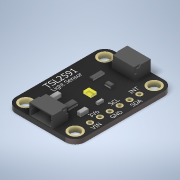
# Autodesk Inventor part: TSL2591
Saved by Autodesk Inventor 2020 (Build 240168000, 168)
## iProperties
Created: 2021-03-24
Part Number: TSL2591
Material: Polyéthylène, densité élevée
Document SubType Name: Modeling
Designer: Charles
Density: 0.952 g/cm^3
Appearance: Lustré - Noir
Author: Charles
Autodesk Inventor part; units mm, degrees
(part 1 of 2)
ref_plane "YZ Plane" through (0, 0, 0) normal (1, 0, 0) x (0, 1, 0)
ref_plane "XZ Plane" through (0, 0, 0) normal (0, 1, 0) x (-1, 0, 0)
ref_plane "XY Plane" through (0, 0, 0) normal (0, 0, 1) x (1, 0, 0)
sketch "Esquisse1" plane through (0, 0, 0) normal (0, 1, 0) x (-1, 0, 0)
  line L0 (0, 0) -> (17.78, 0)
  line L1 (17.78, 0) -> (17.78, -25.4)
  line L2 (17.78, -25.4) -> (0, -25.4)
  line L3 (0, -25.4) -> (0, 0)
  dimension "d0" = 25.4
  dimension "d1" = 17.78
  constraints: 8 end point, 2 parallel, 1 horizontal, 1 perpendicular
  measures "d0" distance of L2.end L0.start
  measures "d1" distance of L1.end L2.end
extrude "Extrusion1" add sketch "Esquisse1" along normal blind 1.2
sketch "Esquisse2" plane through (0, 1.2, 0) normal (0, 1, 0) x (1, 0, 0)
  line L0 (0, 0) -> (0, 25.4) projected
  line L1 (0, 25.4) -> (-17.78, 25.4) projected
  line L2 (0, 0) -> (-17.78, 0)
  line L3 (-17.78, 0) -> (-17.78, 25.4)
  line L4 (-17.78, 25.4) -> (0, 25.4)
  line L5 (0, 25.4) -> (0, 0)
  line L6 (-15.24, 22.86) -> (-15.24, 2.54)
  line L7 (-15.24, 2.54) -> (-2.54, 2.54)
  line L8 (-2.54, 2.54) -> (-2.54, 22.86)
  line L9 (-2.54, 22.86) -> (-15.24, 22.86)
  dimension "d4" = 2.54
  constraints: 16 end point, 4 coincident, 4 parallel, 2 perpendicular, 1 horizontal, 3 other
  measures "d4" distance between parallel lines of L3 L6
hole "Perçage1" at (-15.24, 1.2, -2.54) at (-2.54, 1.2, -2.54) at (-15.24, 1.2, -22.86) at (-2.54, 1.2, -22.86) direction (0, -1, 0) diameter 2.54 end through all
fillet "Congé1" radius 2.54 4 edges at (-17.78, 0.6, 0) (0, 0.6, 0) (0, 0.6, -25.4) (-17.78, 0.6, -25.4)
sketch "Esquisse3" plane through (0, 1.2, 0) normal (0, 1, 0) x (1, 0, 0)
  circle A0 centre (-2.54, 2.54) radius 1.27 projected
  circle A1 centre (-2.54, 22.86) radius 1.27 projected
  line L0 (-2.54, 2.54) -> (-2.54, 22.86)
  circle A2 centre (-2.54, 6.35) radius 0.4
  line L1 (-2.54, 3.81) -> (-4.1087, 3.81)
  circle A3 centre (-2.54, 8.89) radius 0.4
  circle A4 centre (-2.54, 11.43) radius 0.4
  circle A5 centre (-2.54, 13.97) radius 0.4
  circle A6 centre (-2.54, 16.51) radius 0.4
  circle A7 centre (-2.54, 19.05) radius 0.4
  line L2 (-2.54, 21.59) -> (-3.81, 21.59)
  circle A8 centre (-2.54, 6.35) radius 0.75
  circle A9 centre (-2.54, 2.54) radius 1.77
  circle A10 centre (-2.54, 22.86) radius 1.77
  circle A11 centre (-15.24, 22.86) radius 1.27 projected
  circle A12 centre (-15.24, 22.86) radius 1.77
  circle A13 centre (-15.24, 2.54) radius 1.27 projected
  circle A14 centre (-15.24, 2.54) radius 1.77
  circle A15 centre (-2.54, 8.89) radius 0.75
  circle A16 centre (-2.54, 11.43) radius 0.75
  circle A17 centre (-2.54, 13.97) radius 0.75
  circle A18 centre (-2.54, 16.51) radius 0.75
  circle A19 centre (-2.54, 19.05) radius 0.75
  point P0 (0, 0)
  dimension "d13" = 0.8
  dimension "d14" = 2.54
  dimension "d17" = 2.54
  dimension "d23" = 1.5
  dimension "d24" = 3.54
  dimension "d27" = 2.54
  constraints: 16 centre point, 6 end point, 5 coincident, 4 horizontal, 3 point on line, 3 vertical, 2 vertical alignment, 22 other
  measures "d13" diameter of A2
  measures "d14" distance of L1.start A2.centre
  measures "d17" distance of A2.centre A3.centre
  measures "d23" diameter of A8
  measures "d24" diameter of A9
  measures "d27" distance of A8.centre A15.centre
extrude "Extrusion2" cut sketch "Esquisse3" against normal blind 1.2 contours A2 L0 | L0 A2 | A3 L0 | L0 A3 | A4 L0 | L0 A4 | A5 L0 | L0 A5 | A6 L0 | L0 A6 | A7 L0 | L0 A7
extrude "Extrusion3" cut sketch "Esquisse3" against normal blind 0.01 contours L0 A9 L1 | L1 A9 L0 | L2 A10 L0 | L0 A10 L2 | A8 L0 A2 | L0 A2 A8 | A15 L0 A3 | L0 A3 A15 | A16 L0 A4 | L0 A4 A16 | A17 L0 A5 | L0 A5 A17 | A18 L0 A6 | L0 A6 A18 | A19 L0 A7 | L0 A7 A19 | A12 | A14
sketch "Esquisse4" plane through (0, 0, 0) normal (0, -1, 0) x (1, 0, 0)
  circle A0 centre (-2.54, -2.54) radius 1.27 projected
  circle A1 centre (-2.54, -2.54) radius 1.77
  circle A2 centre (-2.54, -6.35) radius 0.4 projected
  circle A3 centre (-2.54, -6.35) radius 0.75
  circle A4 centre (-15.24, -2.54) radius 1.27 projected
  circle A5 centre (-15.24, -2.54) radius 1.77
  circle A6 centre (-15.24, -22.86) radius 1.27 projected
  circle A7 centre (-15.24, -22.86) radius 1.77
  circle A8 centre (-2.54, -22.86) radius 1.27 projected
  circle A9 centre (-2.54, -22.86) radius 1.77
  circle A10 centre (-2.54, -8.89) radius 0.4 projected
  circle A11 centre (-2.54, -8.89) radius 0.75
  circle A12 centre (-2.54, -11.43) radius 0.4 projected
  circle A13 centre (-2.54, -11.43) radius 0.75
  circle A14 centre (-2.54, -13.97) radius 0.4 projected
  circle A15 centre (-2.54, -13.97) radius 0.75
  circle A16 centre (-2.54, -16.51) radius 0.4 projected
  circle A17 centre (-2.54, -16.51) radius 0.75
  circle A18 centre (-2.54, -19.05) radius 0.4 projected
  circle A19 centre (-2.54, -19.05) radius 0.75
  point P0 (0, 0)
  constraints: 10 centre point, 10 coincident
extrude "Extrusion4" cut sketch "Esquisse4" against normal blind 0.01
sketch "Esquisse5" plane through (0, 1.2, 0) normal (0, 1, 0) x (1, 0, 0)
  line L0 (-15.24, 0) -> (-2.54, 0) projected
  line L1 (-8.89, 0) -> (-11.89, 0)
  line L2 (-11.89, 0) -> (-11.89, 4.1)
  line L3 (-11.89, 4.1) -> (-5.89, 4.1)
  line L4 (-5.89, 4.1) -> (-5.89, 0)
  line L5 (-8.89, 0) -> (-5.89, 0)
  line L6 (0, 2.54) -> (0, 22.86) projected
  line L7 (0, 12.7) -> (-5.1683, 12.7)
  line L8 (-8.89, 25.4) -> (-11.89, 25.4)
  line L9 (-11.89, 25.4) -> (-11.89, 21.3)
  line L10 (-11.89, 21.3) -> (-5.89, 21.3)
  line L11 (-5.89, 21.3) -> (-5.89, 25.4)
  line L12 (-8.89, 25.4) -> (-5.89, 25.4)
  point P0 (0, 0)
  dimension "d38" = 3
  dimension "d39" = 4.1
  dimension "d40" = 6
  constraints: 22 end point, 5 symmetric about line, 4 perpendicular, 2 midpoint, 2 point on line, 1 horizontal
  measures "d38" distance of L1.start L1.end
  measures "d39" distance of L1.end L2.end
  measures "d40" distance of L2.end L3.end
extrude "Extrusion5" add sketch "Esquisse5" along normal blind 3
sketch "Esquisse6" plane through (-5.89, 1.2, 0) normal (1, 0, 0) x (0, 0, -1)
  line L0 (4.1, 0) -> (4.1, 3) projected
  line L1 (4.1, 3) -> (2.6, 3)
  line L2 (4.1, 3) -> (0, 3) projected
  line L3 (2.6, 3) -> (2.6, 2.5)
  line L4 (2.6, 2.5) -> (3.6, 2.5)
  line L5 (3.6, 2.5) -> (3.6, 1.5)
  line L6 (3.6, 1.5) -> (4.1, 1.5)
  line L7 (4.1, 3) -> (4.1, 1.5)
  line L8 (2.6, 2.5) -> (2.9, 2.5)
  line L9 (2.9, 2.5) -> (2.6, 3)
  line L10 (2.54, 0) -> (22.86, 0) projected
  line L11 (12.7, 0) -> (12.7, 2)
  line L12 (21.3, 3) -> (22.8, 3)
  line L13 (22.8, 3) -> (22.8, 2.5)
  line L14 (22.8, 2.5) -> (21.8, 2.5)
  line L15 (21.8, 2.5) -> (21.8, 1.5)
  line L16 (21.8, 1.5) -> (21.3, 1.5)
  line L17 (21.3, 3) -> (21.3, 1.5)
  line L18 (22.8, 2.5) -> (22.5, 2.5)
  line L19 (22.5, 2.5) -> (22.8, 3)
  point P0 (0, -1.2)
  dimension "d43" = 1.5
  dimension "d44" = 0.5
  dimension "d45" = 1
  dimension "d46" = 1
  dimension "d47" = 0.3
  constraints: 34 end point, 7 symmetric about line, 3 point on line, 2 midpoint, 2 perpendicular, 2 vertical, 1 collinear
  measures "d43" distance of L0.end L1.end
  measures "d44" distance of L1.end L3.end
  measures "d45" distance of L3.end L4.end
  measures "d46" distance of L4.end L5.end
  measures "d47" distance of L3.end L8.end
extrude "Extrusion6" cut sketch "Esquisse6" against normal blind 0.3 contours L6 L5 L4 L9 L1 L0 | L12 L19 L14 L15 L16 L17
sketch "Esquisse8" plane through (-11.89, 1.2, -25.4) normal (-1, 0, 0) x (0, 0, 1)
  line L0 (4.1, 3) -> (2.6, 3) projected
  line L1 (4.1, 3) -> (2.6, 3)
  line L2 (2.6, 3) -> (2.9, 2.5) projected
  line L3 (2.6, 3) -> (2.9, 2.5)
  line L4 (2.9, 2.5) -> (3.6, 2.5)
  line L5 (3.6, 2.5) -> (3.6, 1.5) projected
  line L6 (3.6, 2.5) -> (3.6, 1.5)
  line L7 (3.6, 1.5) -> (4.1, 1.5) projected
  line L8 (3.6, 1.5) -> (4.1, 1.5)
  line L9 (4.1, 1.5) -> (4.1, 3) projected
  line L10 (4.1, 1.5) -> (4.1, 3)
  point P0 (25.4, -1.2)
  constraints: 12 end point, 3 collinear, 1 horizontal, 1 parallel, 1 perpendicular
extrude "Extrusion7" cut sketch "Esquisse8" against normal blind 0.3
sketch "Esquisse9" plane through (-11.89, 1.2, -4.1) normal (-1, 0, 0) x (0, 0, 1)
  line L0 (0, 3) -> (1.5, 3)
  line L1 (0, 3) -> (4.1, 3) projected
  line L2 (1.5, 3) -> (1.5, 2.5)
  line L3 (0.5, 2.5) -> (1.2, 2.5) projected
  line L4 (1.5, 2.5) -> (0.5, 2.5)
  line L5 (0.5, 1.5) -> (0.5, 2.5) projected
  line L6 (0.5, 2.5) -> (0.5, 1.5)
  line L7 (0, 1.5) -> (0.5, 1.5) projected
  line L8 (0.5, 1.5) -> (0, 1.5)
  line L9 (0, 1.5) -> (0, 3)
  line L10 (1.2, 2.5) -> (1.5, 3) projected
  line L11 (1.2, 2.5) -> (1.5, 3)
  point P0 (4.1, -1.2)
  dimension "d55" = 1.5
  dimension "d56" = 0.5
  constraints: 14 end point, 3 collinear, 2 perpendicular, 1 point on line
  measures "d55" distance of L0.start L0.end
  measures "d56" distance of L0.end L2.end
extrude "Extrusion8" cut sketch "Esquisse9" against normal blind 0.3 contours L0 L10 L3 L5 L7 L9
sketch "Esquisse10" plane through (0, 4.2, 0) normal (0, 1, 0) x (1, 0, 0)
  line L0 (-2.54, 25.4) -> (-5.89, 25.4) projected
  line L1 (-11.89, 21.3) -> (-11.89, 25.4) projected
  line L2 (-5.89, 25.4) -> (-11.89, 25.4)
  line L3 (-11.89, 25.4) -> (-11.89, 25.3)
  line L4 (-11.89, 25.3) -> (-5.89, 25.3)
  line L5 (-5.89, 25.3) -> (-5.89, 25.4)
  line L6 (-5.89, 0) -> (-2.54, 0) projected
  line L7 (-11.89, 2.6) -> (-11.89, 0) projected
  line L8 (-5.89, 0) -> (-11.89, 0)
  line L9 (-11.89, 0) -> (-11.89, 0.1)
  line L10 (-11.89, 0.1) -> (-5.89, 0.1)
  line L11 (-5.89, 0.1) -> (-5.89, 0)
  point P0 (0, 0)
  dimension "d59" = 0.1
  dimension "d60" = 0.1
  constraints: 16 end point, 4 parallel, 2 horizontal, 2 perpendicular, 2 point on line
  measures "d59" distance of L3.end L2.end
  measures "d60" distance of L8.end L9.end
extrude "Extrusion9" cut sketch "Esquisse10" against normal blind 3
sketch "Esquisse11" plane through (-5.89, 4.2, -25.3) normal (0, 0, -1) x (-1, 0, 0)
  line L0 (0.4, -1.5) -> (5.6, -1.5)
  line L1 (5.6, -1.5) -> (5.6, -2.85)
  line L2 (5.6, -2.85) -> (0.4, -2.85)
  line L3 (0.4, -2.85) -> (0.4, -1.5)
  line L4 (-3.35, -3) -> (9.35, -3) projected
  line L5 (6, 0) -> (6, -3) projected
  line L6 (0, -3) -> (0, 0) projected
  line L7 (5.8, -1.2) -> (0.2, -1.2)
  line L8 (0.2, -1.2) -> (0.2, -1.5)
  line L9 (0.2, -1.5) -> (5.8, -1.5)
  line L10 (5.8, -1.5) -> (5.8, -1.2)
  line L11 (0.4, -1.2) -> (5.6, -1.2)
  line L12 (5.6, -1.2) -> (5.6, -0.2793)
  line L13 (5.6, -0.2793) -> (0.4, -0.2793)
  line L14 (0.4, -0.2793) -> (0.4, -1.2)
  line L15 (0.3, 0) -> (0.3, -1.5) projected
  line L16 (0.4, -1.2) -> (0.4, -1.5)
  line L17 (5.6, -1.2) -> (5.6, -1.5)
  point P0 (-5.89, -4.2)
  point P1 (0.4, -1.5)
  point P2 (5.6, -1.2)
  dimension "d63" = 0.15
  dimension "d64" = 0.4
  dimension "d65" = 0.4
  dimension "d66" = 1.5
  dimension "d67" = 0.2
  dimension "d68" = 0.2
  dimension "d69" = 0.3
  dimension "d70" = 0.4
  dimension "d71" = 0.4
  constraints: 28 end point, 6 parallel, 3 horizontal, 3 perpendicular, 2 point on line
  measures "d63" distance between parallel lines of L4 L2
  measures "d64" distance between parallel lines of L5 L1
  measures "d65" distance between parallel lines of L6 L3
  measures "d66" distance between parallel lines of L4 L0
  measures "d67" distance between parallel lines of L5 L10
  measures "d68" distance between parallel lines of L6 L8
  measures "d69" distance between parallel lines of L0 L7
  measures "d70" distance between parallel lines of L5 L12
  measures "d71" distance between parallel lines of L6 L14
extrude "Extrusion10" cut sketch "Esquisse11" against normal blind 3.5 contours L16 L7 L17 L0 | L0 L1 L2 L3 | L14 L13 L12 L7
extrude "Extrusion11" cut sketch "Esquisse11" against normal blind 3 contours L9 L15 L7 L16 | L17 L7 L10 L9 | L9 L8 L7 L15
sketch "Esquisse12" plane through (-5.89, 4.2, -21.8) normal (0, 0, -1) x (-1, 0, 0)
  line L0 (0.2, -1.2) -> (0.4, -1.2) projected
  line L1 (0.4, -1.2) -> (1.5, -1.2)
  circle A0 centre (1.5, -1.2) radius 0.075
  circle A1 centre (2.5, -1.2) radius 0.075
  circle A2 centre (3.5, -1.2) radius 0.075
  circle A3 centre (4.5, -1.2) radius 0.075
  line L2 (5.6, -0.2793) -> (5.6, -1.2) projected
  point P0 (-5.89, -4.2)
  dimension "d76" = 1.1
  dimension "d77" = 0.15
  dimension "d80" = 1
  dimension "d85" = 1.1
  constraints: 4 centre point, 2 end point, 2 horizontal, 1 coincident, 6 other
  measures "d76" distance of L0.end L1.end
  measures "d77" diameter of A0
  measures "d80" distance of A0.centre A1.centre
  measures "d85" distance from line of L2 A3.centre
extrude "Extrusion12" add sketch "Esquisse12" along normal blind 2.5
chamfer "Chanfrein1" distance 0.075 distance2 0.25 1 edges at (-7.315, 3, -24.3) measured on face at (-7.3698, 2.9853, -24.3)
chamfer "Chanfrein2" distance 0.075 distance2 0.25 1 edges at (-9.315, 3, -24.3) measured on face at (-9.415, 3, -24.3)
chamfer "Chanfrein3" distance 0.075 distance2 0.25 1 edges at (-8.315, 3, -24.3) measured on face at (-8.365, 3, -24.3)
chamfer "Chanfrein4" distance 0.075 distance2 0.25 1 edges at (-10.315, 3, -24.3) measured on face at (-10.3977, 2.9762, -24.3)
sketch "Esquisse13" plane through (-11.89, 4.2, -0.1) normal (0, 0, 1) x (1, 0, 0)
  line L0 (0.4, -0.2793) -> (0.4, -2.85) projected
  line L1 (5.6, -2.85) -> (5.6, -0.2793) projected
  line L2 (0.4, -2.85) -> (5.6, -2.85)
  line L3 (5.6, -2.85) -> (5.6, -0.2793)
  line L4 (5.6, -0.2793) -> (0.4, -0.2793)
  line L5 (0.4, -0.2793) -> (0.4, -2.85)
  line L6 (-3.35, -3) -> (9.35, -3) projected
  line L7 (0.2, -1.2) -> (0.2, -1.5) projected
  line L8 (0.2, -1.2) -> (5.8, -1.2)
  line L9 (5.8, -1.2) -> (5.8, -1.5)
  line L10 (5.8, -1.5) -> (0.2, -1.5)
  line L11 (0.2, -1.5) -> (0.2, -1.2)
  point P0 (11.89, -4.2)
  point P1 (5.6, -1.2)
  point P2 (5.6, -1.5)
  point P3 (0.4, -1.5)
  point P4 (0.4, -1.2)
  dimension "d100" = 0.15
  constraints: 16 end point, 4 parallel, 2 horizontal, 2 perpendicular
  measures "d100" distance between parallel lines of L6 L2
extrude "Extrusion13" cut sketch "Esquisse13" against normal blind 3.5 contours L4 L1 L8 L0 | L8 L1 L10 L0 | L10 L1 L2 L0
extrude "Extrusion14" cut sketch "Esquisse13" against normal blind 3 contours L0 L10 L7 L8 | L8 L9 L10 L1
sketch "Esquisse14" plane through (-11.89, 4.2, -3.6) normal (0, 0, 1) x (1, 0, 0)
  line L0 (0.4, -1.2) -> (1.5, -1.2)
  circle A0 centre (1.5, -1.2) radius 0.075
  circle A1 centre (2.5, -1.2) radius 0.075
  circle A2 centre (3.5, -1.2) radius 0.075
  circle A3 centre (4.5, -1.2) radius 0.075
  point P0 (11.89, -4.2)
  dimension "d105" = 1.1
  dimension "d106" = 0.15
  dimension "d109" = 1
  constraints: 4 centre point, 2 end point, 2 horizontal, 1 coincident, 6 other
  measures "d105" distance of L0.start L0.end
  measures "d106" diameter of A0
  measures "d109" distance of A0.centre A1.centre
extrude "Extrusion15" add sketch "Esquisse14" along normal blind 2.5
chamfer "Chanfrein5" distance 0.075 distance2 0.25 1 edges at (-10.465, 3, -1.1) measured on face at (-10.3977, 2.9762, -1.1)
chamfer "Chanfrein6" distance 0.075 distance2 0.25 1 edges at (-9.465, 3, -1.1) measured on face at (-9.415, 3, -1.1)
chamfer "Chanfrein7" distance 0.075 distance2 0.25 1 edges at (-8.465, 3, -1.1) measured on face at (-8.365, 3, -1.1)
chamfer "Chanfrein8" distance 0.075 distance2 0.25 1 edges at (-7.465, 3, -1.1) measured on face at (-7.3823, 2.9762, -1.1)
sketch "Esquisse15" plane through (0, 1.2, 0) normal (0, 1, 0) x (1, 0, 0)
  circle A0 centre (-15.24, 2.54) radius 1.27 projected
  circle A1 centre (-2.54, 22.86) radius 1.27 projected
  line L0 (-2.54, 22.86) -> (-15.24, 2.54)
  circle A2 centre (-2.54, 2.54) radius 1.27 projected
  circle A3 centre (-15.24, 22.86) radius 1.27 projected
  line L1 (-2.54, 2.54) -> (-15.24, 22.86)
  line L2 (-7.89, 13.45) -> (-9.89, 13.45)
  line L3 (-9.89, 13.45) -> (-9.89, 11.95)
  line L4 (-9.89, 11.95) -> (-7.89, 11.95)
  line L5 (-7.89, 11.95) -> (-7.89, 13.45)
  line L6 (-7.89, 13.45) -> (-9.89, 11.95) construction
  line L7 (-9.89, 13.45) -> (-7.89, 11.95) construction
  line L8 (-6.19, 4.1) -> (-11.59, 4.1) projected
  line L9 (-8.89, 4.1) -> (-8.89, 21.3)
  line L10 (-11.59, 21.3) -> (-6.19, 21.3) projected
  line L11 (-8.89, 4.1) -> (-8.89, 6.1)
  line L12 (-8.89, 6.1) -> (-9.39, 6.1)
  line L13 (-9.39, 6.1) -> (-9.39, 8.6)
  line L14 (-9.39, 8.6) -> (-7.89, 8.6)
  line L15 (-7.89, 8.6) -> (-7.89, 6.1)
  line L16 (-7.89, 6.1) -> (-8.89, 6.1)
  line L17 (-11.89, 0.1) -> (-11.89, 4.1) projected
  line L18 (-11.89, 4.1) -> (-11.89, 8.7)
  line L19 (-9.39, 7.35) -> (-11.89, 7.35)
  line L20 (-11.89, 7.35) -> (-11.89, 8.35)
  line L21 (-11.89, 8.35) -> (-12.89, 8.35)
  line L22 (-12.89, 8.35) -> (-12.89, 6.35)
  line L23 (-12.89, 6.35) -> (-11.89, 6.35)
  line L24 (-11.89, 4.1) -> (-5.89, 4.1) projected
  line L25 (-5.89, 4.1) -> (-5.89, 7.35)
  line L26 (-5.89, 7.35) -> (-5.89, 8.35)
  line L27 (-5.89, 8.35) -> (-4.89, 8.35)
  line L28 (-4.89, 8.35) -> (-4.89, 6.35)
  line L29 (-4.89, 6.35) -> (-5.89, 6.35)
  line L30 (-5.89, 8.35) -> (-5.89, 11.95)
  line L31 (-5.89, 11.95) -> (-7.89, 11.95)
  line L32 (-5.89, 11.95) -> (-5.89, 12.7)
  line L33 (-5.89, 12.7) -> (-5.29, 12.7)
  line L34 (-5.29, 12.7) -> (-5.29, 11.2)
  line L35 (-5.29, 11.2) -> (-5.89, 11.2)
  line L36 (-8.89, 12.7) -> (-8.89, 21.3)
  line L37 (-8.89, 17) -> (-8.89, 17.5)
  line L38 (-8.89, 17.5) -> (-7.39, 17.5)
  line L39 (-7.39, 17.5) -> (-7.39, 16.5)
  line L40 (-7.39, 16.5) -> (-8.89, 16.5)
  line L41 (-11.89, 21.3) -> (-11.89, 16)
  line L42 (-8.89, 16.5) -> (-8.89, 16)
  line L43 (-8.89, 16) -> (-12.39, 16)
  line L44 (-11.89, 16) -> (-11.39, 16)
  line L45 (-11.39, 16) -> (-11.39, 19)
  line L46 (-11.39, 19) -> (-12.39, 19)
  line L47 (-12.39, 19) -> (-12.39, 16)
  point P0 (0, 0)
  dimension "d130" = 2
  dimension "d131" = 1.5
  dimension "d132" = 2
  dimension "d133" = 0.5
  dimension "d134" = 2.5
  dimension "d135" = 1.5
  dimension "d136" = 1
  dimension "d137" = 1
  dimension "d139" = 2
  dimension "d140" = 1
  dimension "d142" = 3.25
  dimension "d143" = 1
  dimension "d144" = 2
  dimension "d145" = 0.6
  dimension "d146" = 1.5
  dimension "d147" = 0.5
  dimension "d148" = 1
  dimension "d149" = 1.5
  dimension "d150" = 0.5
  dimension "d151" = 0.5
  dimension "d152" = 3
  dimension "d153" = 1
  constraints: 90 end point, 21 perpendicular, 13 point on line, 7 midpoint, 7 vertical, 2 parallel, 1 collinear, 1 horizontal
  measures "d130" distance of L4.end L3.end
  measures "d131" distance of L3.end L2.end
  measures "d132" distance of L9.start L11.end
  measures "d133" distance of L11.end L12.end
  measures "d134" distance of L12.end L13.end
  measures "d135" distance of L13.end L14.end
  measures "d136" distance of L19.end L20.end
  measures "d137" distance of L20.end L21.end
  measures "d139" distance from line of L21 L22.end
  measures "d140" distance of L26.end L27.end
  measures "d142" distance of L24.end L25.end
  measures "d143" distance of L25.end L26.end
  measures "d144" distance between parallel lines of L27 L29
  measures "d145" distance of L32.end L33.end
  measures "d146" distance of L33.end L34.end
  measures "d147" distance of L37.start L37.end
  measures "d148" distance of L38.end L39.end
  measures "d149" distance of L37.end L38.end
  measures "d150" distance of L40.end L42.end
  measures "d151" distance of L41.end L44.end
  measures "d152" distance of L44.end L45.end
  measures "d153" distance of L45.end L46.end
extrude "Extrusion16" add sketch "Esquisse15" along normal blind 0.9 contours L18 L23 L0 | L0 L23 L22 L21 L18 | L26 L27 L28 L29 L1 | L1 L29 L25 L26
extrude "Extrusion17" add sketch "Esquisse15" along normal blind 0.7 contours L14 L15 L16 L9 | L9 L12 L13 L14
extrude "Extrusion18" add sketch "Esquisse15" along normal blind 0.6 contours L2 L5 L4 L1 L0 | L0 L9 L2 | L9 L4 L0 | L0 L4 L3 L2 L1 | L1 L4 L9 | L1 L2 L9 | L32 L33 L34 L35 L30 | L9 L38 L39 L40
extrude "Extrusion19" add sketch "Esquisse15" along normal blind 0.4 contours L45 L43 L41 L1 | L1 L41 L46 L45 | L41 L43 L47 L1 | L1 L47 L46 L41
chamfer "Chanfrein9" distance 0.075 distance2 0.25 1 edges at (-9.39, 1.9, -7.35) measured on face at (-8.89, 1.9, -7.7667)
chamfer "Chanfrein10" distance 0.075 distance2 0.25 1 edges at (-7.89, 1.9, -7.35) measured on face at (-8.84, 1.9, -7.7667)
chamfer "Chanfrein11" distance 0.05 distance2 0.25 1 edges at (-8.14, 1.8, -16.5) measured on face at (-8.39, 1.8, -17.1667)
chamfer "Chanfrein12" distance 0.05 distance2 0.25 1 edges at (-8.14, 1.8, -17.5) measured on face at (-8.39, 1.8, -17.1833)
fillet "Congé2" radius 0.05 12 edges at (-5.29, 1.8, -11.95) (-5.59, 1.8, -12.7) (-5.89, 1.8, -11.95) (-5.59, 1.8, -11.2) (-4.89, 2.1, -7.35) (-5.39, 2.1, -8.35) (-5.89, 2.1, -7.35) (-5.39, 2.1, -6.35) (-11.89, 2.1, -7.35) (-12.39, 2.1, -6.35) (-12.89, 2.1, -7.35) (-12.39, 2.1, -8.35)
sketch "Esquisse16" plane through (0, 1.2, 0) normal (0, 1, 0) x (1, 0, 0)
  line L0 (-17.0244, 8.4742) -> (-17.0244, 16.4163) construction
  line L1 (-17.0244, 16.4163) -> (-15.3143, 16.4163) construction
  line L2 (-15.3143, 16.4163) -> (-15.3143, 8.4742) construction
  line L3 (-15.3143, 8.4742) -> (-17.0244, 8.4742) construction
  line L4 (-15.1503, 8.6002) -> (-15.1503, 17.1987) construction
  line L5 (-15.1503, 17.1987) -> (-14.0322, 17.1987) construction
  line L6 (-14.0322, 17.1987) -> (-14.0322, 8.6002) construction
  line L7 (-14.0322, 8.6002) -> (-15.1503, 8.6002) construction
  line L8 (-15.4928, 8.9762) -> (-16.8153, 8.9762)
  line L9 (-16.8153, 8.9762) -> (-16.8153, 8.473)
  line L10 (-16.8153, 8.473) -> (-16.9928, 8.473)
  line L11 (-16.9928, 8.473) -> (-16.9928, 9.6788)
  line L12 (-16.9928, 9.6788) -> (-16.8153, 9.6788)
  line L13 (-16.8153, 9.6788) -> (-16.8153, 9.1756)
  line L14 (-16.8153, 9.1756) -> (-15.4928, 9.1756)
  line L15 (-15.4928, 9.1756) -> (-15.4928, 8.9762)
  spline S0 degree 2 poles (-15.466, 10.2489) (-15.466, 10.086) (-15.5341, 9.8575) (-15.5827, 9.7566) knots 0 0 0 1 2 2 2
  line L16 (-15.5827, 9.7566) -> (-15.8331, 9.7566)
  line L17 (-15.8331, 9.7566) -> (-15.8331, 9.7712)
  spline S1 degree 2 poles (-15.8331, 9.7712) (-15.7407, 9.8696) (-15.6386, 10.1188) (-15.6386, 10.2343) knots 0 0 0 1 2 2 2
  spline S2 degree 2 poles (-15.6386, 10.2343) (-15.6386, 10.3996) (-15.776, 10.5686) (-15.889, 10.5686) knots 0 0 0 1 2 2 2
  spline S3 degree 2 poles (-15.889, 10.5686) (-15.979, 10.5686) (-16.0908, 10.4799) (-16.1188, 10.3838) knots 0 0 0 1 2 2 2
  spline S4 degree 2 poles (-16.1188, 10.3838) (-16.1382, 10.3145) (-16.165, 10.1991) (-16.1868, 10.1128) knots 0 0 0 1 2 2 2
  spline S5 degree 2 poles (-16.1868, 10.1128) (-16.2075, 10.035) (-16.2695, 9.9122) (-16.3193, 9.8648) knots 0 0 0 1 2 2 2
  spline S6 degree 2 poles (-16.3193, 9.8648) (-16.3692, 9.8186) (-16.5029, 9.7675) (-16.5904, 9.7675) knots 0 0 0 1 2 2 2
  spline S7 degree 2 poles (-16.5904, 9.7675) (-16.7727, 9.7675) (-17.0195, 10.052) (-17.0195, 10.272) knots 0 0 0 1 2 2 2
  spline S8 degree 2 poles (-17.0195, 10.272) (-17.0195, 10.3984) (-16.9697, 10.6221) (-16.9222, 10.7181) knots 0 0 0 1 2 2 2
  line L18 (-16.9222, 10.7181) -> (-16.684, 10.7181)
  line L19 (-16.684, 10.7181) -> (-16.684, 10.7035)
  spline S9 degree 2 poles (-16.684, 10.7035) (-16.7496, 10.6318) (-16.8469, 10.4081) (-16.8469, 10.2854) knots 0 0 0 1 2 2 2
  spline S10 degree 2 poles (-16.8469, 10.2854) (-16.8469, 10.1468) (-16.7168, 9.9754) (-16.6111, 9.9754) knots 0 0 0 1 2 2 2
  spline S11 degree 2 poles (-16.6111, 9.9754) (-16.5163, 9.9754) (-16.4032, 10.0763) (-16.3777, 10.1711) knots 0 0 0 1 2 2 2
  spline S12 degree 2 poles (-16.3777, 10.1711) (-16.3607, 10.2343) (-16.3169, 10.4179) (-16.2987, 10.4786) knots 0 0 0 1 2 2 2
  spline S13 degree 2 poles (-16.2987, 10.4786) (-16.2513, 10.633) (-16.0604, 10.7764) (-15.9206, 10.7764) knots 0 0 0 1 2 2 2
  spline S14 degree 2 poles (-15.9206, 10.7764) (-15.8319, 10.7764) (-15.6617, 10.7047) (-15.6022, 10.6403) knots 0 0 0 1 2 2 2
  spline S15 degree 2 poles (-15.6022, 10.6403) (-15.5365, 10.5686) (-15.466, 10.3863) (-15.466, 10.2489) knots 0 0 0 1 2 2 2
  line L20 (-15.4928, 11.8486) -> (-15.4928, 10.9794)
  line L21 (-15.4928, 10.9794) -> (-16.9928, 10.9794)
  line L22 (-16.9928, 10.9794) -> (-16.9928, 11.1788)
  line L23 (-16.9928, 11.1788) -> (-15.6702, 11.1788)
  line L24 (-15.6702, 11.1788) -> (-15.6702, 11.8486)
  line L25 (-15.6702, 11.8486) -> (-15.4928, 11.8486)
  line L26 (-15.4928, 12.8879) -> (-15.4928, 11.9628)
  line L27 (-15.4928, 11.9628) -> (-15.7055, 11.9628)
  spline S16 degree 2 poles (-15.7055, 11.9628) (-15.7991, 12.0625) (-15.9729, 12.24) (-16.0665, 12.3251) knots 0 0 0 1 2 2 2
  spline S17 degree 2 poles (-16.0665, 12.3251) (-16.2549, 12.4965) (-16.481, 12.6217) (-16.6013, 12.6217) knots 0 0 0 1 2 2 2
  spline S18 degree 2 poles (-16.6013, 12.6217) (-16.6646, 12.6217) (-16.7594, 12.5828) (-16.7898, 12.5475) knots 0 0 0 1 2 2 2
  spline S19 degree 2 poles (-16.7898, 12.5475) (-16.8201, 12.5123) (-16.8505, 12.4199) (-16.8505, 12.364) knots 0 0 0 1 2 2 2
  spline S20 degree 2 poles (-16.8505, 12.364) (-16.8505, 12.3105) (-16.8238, 12.2011) (-16.8031, 12.1512) knots 0 0 0 1 2 2 2
  spline S21 degree 2 poles (-16.8031, 12.1512) (-16.7861, 12.1087) (-16.7375, 12.0297) (-16.7205, 12.0054) knots 0 0 0 1 2 2 2
  line L28 (-16.7205, 12.0054) -> (-16.7205, 11.9944)
  line L29 (-16.7205, 11.9944) -> (-16.9344, 11.9944)
  spline S22 degree 2 poles (-16.9344, 11.9944) (-16.9648, 12.0564) (-17.0244, 12.2789) (-17.0244, 12.3786) knots 0 0 0 1 2 2 2
  spline S23 degree 2 poles (-17.0244, 12.3786) (-17.0244, 12.5888) (-16.8019, 12.8259) (-16.6123, 12.8259) knots 0 0 0 1 2 2 2
  spline S24 degree 2 poles (-16.6123, 12.8259) (-16.5235, 12.8259) (-16.3752, 12.7846) (-16.312, 12.7481) knots 0 0 0 1 2 2 2
  spline S25 degree 2 poles (-16.312, 12.7481) (-16.2464, 12.7116) (-16.1175, 12.6059) (-16.0556, 12.5475) knots 0 0 0 1 2 2 2
  spline S26 degree 2 poles (-16.0556, 12.5475) (-15.9522, 12.4527) (-15.731, 12.2205) (-15.6666, 12.1512) knots 0 0 0 1 2 2 2
  line L30 (-15.6666, 12.1512) -> (-15.6666, 12.8879)
  line L31 (-15.6666, 12.8879) -> (-15.4928, 12.8879)
  spline S27 degree 2 poles (-15.9693, 13.9977) (-15.8611, 13.9977) (-15.6763, 13.9284) (-15.6082, 13.8652) knots 0 0 0 1 2 2 2
  spline S28 degree 2 poles (-15.6082, 13.8652) (-15.5402, 13.802) (-15.4611, 13.6136) (-15.4611, 13.4969) knots 0 0 0 1 2 2 2
  spline S29 degree 2 poles (-15.4611, 13.4969) (-15.4611, 13.3899) (-15.5086, 13.1808) (-15.5462, 13.1042) knots 0 0 0 1 2 2 2
  line L32 (-15.5462, 13.1042) -> (-15.759, 13.1042)
  line L33 (-15.759, 13.1042) -> (-15.759, 13.1188)
  spline S30 degree 2 poles (-15.759, 13.1188) (-15.7419, 13.1419) (-15.6982, 13.2282) (-15.6787, 13.2805) knots 0 0 0 1 2 2 2
  spline S31 degree 2 poles (-15.6787, 13.2805) (-15.6581, 13.3401) (-15.635, 13.4385) (-15.635, 13.5005) knots 0 0 0 1 2 2 2
  spline S32 degree 2 poles (-15.635, 13.5005) (-15.635, 13.5613) (-15.6787, 13.6756) (-15.7261, 13.7169) knots 0 0 0 1 2 2 2
  spline S33 degree 2 poles (-15.7261, 13.7169) (-15.7711, 13.7546) (-15.8902, 13.7935) (-15.9705, 13.7935) knots 0 0 0 1 2 2 2
  spline S34 degree 2 poles (-15.9705, 13.7935) (-16.0507, 13.7935) (-16.1528, 13.7497) (-16.1868, 13.7084) knots 0 0 0 1 2 2 2
  spline S35 degree 2 poles (-16.1868, 13.7084) (-16.2245, 13.6658) (-16.2561, 13.5394) (-16.2561, 13.4628) knots 0 0 0 1 2 2 2
  spline S36 degree 2 poles (-16.2561, 13.4628) (-16.2561, 13.3802) (-16.2306, 13.2161) (-16.2197, 13.1662) knots 0 0 0 1 2 2 2
  line L34 (-16.2197, 13.1662) -> (-16.9928, 13.1662)
  line L35 (-16.9928, 13.1662) -> (-16.9928, 13.9892)
  line L36 (-16.9928, 13.9892) -> (-16.8165, 13.9892)
  line L37 (-16.8165, 13.9892) -> (-16.8165, 13.3595)
  line L38 (-16.8165, 13.3595) -> (-16.4166, 13.3595)
  spline S37 degree 2 poles (-16.4166, 13.3595) (-16.4214, 13.396) (-16.4251, 13.4665) (-16.4251, 13.4957) knots 0 0 0 1 2 2 2
  spline S38 degree 2 poles (-16.4251, 13.4957) (-16.4251, 13.6111) (-16.3874, 13.7704) (-16.3315, 13.8433) knots 0 0 0 1 2 2 2
  spline S39 degree 2 poles (-16.3315, 13.8433) (-16.2756, 13.9175) (-16.1054, 13.9977) (-15.9693, 13.9977) knots 0 0 0 1 2 2 2
  spline S40 degree 2 poles (-16.5053, 14.1727) (-16.6208, 14.1727) (-16.8128, 14.2481) (-16.8821, 14.3137) knots 0 0 0 1 2 2 2
  spline S41 degree 2 poles (-16.8821, 14.3137) (-16.949, 14.3757) (-17.0231, 14.5568) (-17.0231, 14.6492) knots 0 0 0 1 2 2 2
  spline S42 degree 2 poles (-17.0231, 14.6492) (-17.0231, 14.7525) (-16.9539, 14.9203) (-16.8882, 14.9823) knots 0 0 0 1 2 2 2
  spline S43 degree 2 poles (-16.8882, 14.9823) (-16.8056, 15.0601) (-16.5381, 15.1452) (-16.3327, 15.1452) knots 0 0 0 1 2 2 2
  spline S44 degree 2 poles (-16.3327, 15.1452) (-16.1467, 15.1452) (-15.8137, 15.0613) (-15.703, 14.9799) knots 0 0 0 1 2 2 2
  spline S45 degree 2 poles (-15.703, 14.9799) (-15.5864, 14.8935) (-15.4636, 14.6504) (-15.4636, 14.473) knots 0 0 0 1 2 2 2
  spline S46 degree 2 poles (-15.4636, 14.473) (-15.4636, 14.4328) (-15.4721, 14.3417) (-15.4842, 14.3028) knots 0 0 0 1 2 2 2
  line L39 (-15.4842, 14.3028) -> (-15.6775, 14.3028)
  line L40 (-15.6775, 14.3028) -> (-15.6775, 14.3125)
  spline S47 degree 2 poles (-15.6775, 14.3125) (-15.6629, 14.338) (-15.6374, 14.445) (-15.6374, 14.4997) knots 0 0 0 1 2 2 2
  spline S48 degree 2 poles (-15.6374, 14.4997) (-15.6374, 14.6966) (-15.8975, 14.9215) (-16.1382, 14.9373) knots 0 0 0 1 2 2 2
  spline S49 degree 2 poles (-16.1382, 14.9373) (-16.0835, 14.8571) (-16.0337, 14.7112) (-16.0337, 14.6249) knots 0 0 0 1 2 2 2
  spline S50 degree 2 poles (-16.0337, 14.6249) (-16.0337, 14.5422) (-16.0701, 14.4049) (-16.1224, 14.3356) knots 0 0 0 1 2 2 2
  spline S51 degree 2 poles (-16.1224, 14.3356) (-16.1844, 14.2554) (-16.3728, 14.1727) (-16.5053, 14.1727) knots 0 0 0 1 2 2 2
  spline S52 degree 2 poles (-16.3777, 14.9422) (-16.5296, 14.9422) (-16.7217, 14.8863) (-16.774, 14.8364) knots 0 0 0 1 2 2 2
  spline S53 degree 2 poles (-16.774, 14.8364) (-16.8226, 14.7927) (-16.859, 14.7015) (-16.859, 14.648) knots 0 0 0 1 2 2 2
  spline S54 degree 2 poles (-16.859, 14.648) (-16.859, 14.524) (-16.6816, 14.3769) (-16.5138, 14.3769) knots 0 0 0 1 2 2 2
  spline S55 degree 2 poles (-16.5138, 14.3769) (-16.419, 14.3769) (-16.2962, 14.4256) (-16.2525, 14.479) knots 0 0 0 1 2 2 2
  spline S56 degree 2 poles (-16.2525, 14.479) (-16.2209, 14.5179) (-16.2002, 14.614) (-16.2002, 14.6699) knots 0 0 0 1 2 2 2
  spline S57 degree 2 poles (-16.2002, 14.6699) (-16.2002, 14.7343) (-16.2452, 14.8826) (-16.2829, 14.9385) knots 0 0 0 1 2 2 2
  spline S58 degree 2 poles (-16.2829, 14.9385) (-16.2975, 14.9397) (-16.3473, 14.9422) (-16.3777, 14.9422) knots 0 0 0 1 2 2 2
  line L41 (-15.4928, 16.1893) -> (-15.4928, 15.4576)
  line L42 (-15.4928, 15.4576) -> (-15.6459, 15.4576)
  line L43 (-15.6459, 15.4576) -> (-15.6459, 15.7299)
  line L44 (-15.6459, 15.7299) -> (-16.6512, 15.7299)
  line L45 (-16.6512, 15.7299) -> (-16.6512, 15.4576)
  line L46 (-16.6512, 15.4576) -> (-16.7885, 15.4576)
  spline S59 degree 2 poles (-16.7885, 15.4576) (-16.7885, 15.6119) (-16.8761, 15.7578) (-16.9976, 15.7675) knots 0 0 0 1 2 2 2
  line L47 (-16.9976, 15.7675) -> (-16.9976, 15.9231)
  line L48 (-16.9976, 15.9231) -> (-15.6459, 15.9231)
  line L49 (-15.6459, 15.9231) -> (-15.6459, 16.1893)
  line L50 (-15.6459, 16.1893) -> (-15.4928, 16.1893)
  line L51 (-14.1058, 9.2809) -> (-14.1058, 8.7015)
  line L52 (-14.1058, 8.7015) -> (-15.1058, 8.7015)
  line L53 (-15.1058, 8.7015) -> (-15.1058, 8.8344)
  line L54 (-15.1058, 8.8344) -> (-14.2241, 8.8344)
  line L55 (-14.2241, 8.8344) -> (-14.2241, 9.2809)
  line L56 (-14.2241, 9.2809) -> (-14.1058, 9.2809)
  line L57 (-14.1058, 9.5045) -> (-14.1058, 9.3781)
  line L58 (-14.1058, 9.3781) -> (-14.8562, 9.3781)
  line L59 (-14.8562, 9.3781) -> (-14.8562, 9.5045)
  line L60 (-14.8562, 9.5045) -> (-14.1058, 9.5045)
  line L61 (-14.981, 9.5134) -> (-14.981, 9.37)
  line L62 (-14.981, 9.37) -> (-15.1123, 9.37)
  line L63 (-15.1123, 9.37) -> (-15.1123, 9.5134)
  line L64 (-15.1123, 9.5134) -> (-14.981, 9.5134)
  spline S60 degree 2 poles (-13.9858, 9.7169) (-13.9802, 9.7298) (-13.9623, 9.7793) (-13.955, 9.8109) knots 0 0 0 1 2 2 2
  spline S61 degree 2 poles (-13.955, 9.8109) (-13.9461, 9.8457) (-13.9356, 9.9049) (-13.9356, 9.9397) knots 0 0 0 1 2 2 2
  spline S62 degree 2 poles (-13.9356, 9.9397) (-13.9356, 9.9981) (-13.9664, 10.0791) (-13.9939, 10.1018) knots 0 0 0 1 2 2 2
  spline S63 degree 2 poles (-13.9939, 10.1018) (-14.0215, 10.1237) (-14.0936, 10.1407) (-14.1398, 10.1407) knots 0 0 0 1 2 2 2
  line L65 (-14.1398, 10.1407) -> (-14.2054, 10.1407)
  spline S64 degree 2 poles (-14.2054, 10.1407) (-14.1609, 10.0896) (-14.1187, 9.9916) (-14.1187, 9.9178) knots 0 0 0 1 2 2 2
  spline S65 degree 2 poles (-14.1187, 9.9178) (-14.1187, 9.7898) (-14.3092, 9.6382) (-14.4883, 9.6382) knots 0 0 0 1 2 2 2
  spline S66 degree 2 poles (-14.4883, 9.6382) (-14.5815, 9.6382) (-14.7257, 9.6909) (-14.7768, 9.7347) knots 0 0 0 1 2 2 2
  spline S67 degree 2 poles (-14.7768, 9.7347) (-14.8246, 9.7768) (-14.8772, 9.8927) (-14.8772, 9.9543) knots 0 0 0 1 2 2 2
  spline S68 degree 2 poles (-14.8772, 9.9543) (-14.8772, 10.0126) (-14.8497, 10.0977) (-14.8246, 10.1407) knots 0 0 0 1 2 2 2
  line L66 (-14.8246, 10.1407) -> (-14.8562, 10.148)
  line L67 (-14.8562, 10.148) -> (-14.8562, 10.2671)
  line L68 (-14.8562, 10.2671) -> (-14.1917, 10.2671)
  spline S69 degree 2 poles (-14.1917, 10.2671) (-14.0004, 10.2671) (-13.8221, 10.101) (-13.8221, 9.93) knots 0 0 0 1 2 2 2
  spline S70 degree 2 poles (-13.8221, 9.93) (-13.8221, 9.8749) (-13.84, 9.7598) (-13.8546, 9.7104) knots 0 0 0 1 2 2 2
  line L69 (-13.8546, 9.7104) -> (-13.9858, 9.7104)
  line L70 (-13.9858, 9.7104) -> (-13.9858, 9.7169)
  line L71 (-14.3092, 10.1407) -> (-14.7217, 10.1407)
  spline S71 degree 2 poles (-14.7217, 10.1407) (-14.7443, 10.0937) (-14.7638, 10.0143) (-14.7638, 9.9746) knots 0 0 0 1 2 2 2
  spline S72 degree 2 poles (-14.7638, 9.9746) (-14.7638, 9.8789) (-14.6228, 9.7687) (-14.4907, 9.7687) knots 0 0 0 1 2 2 2
  spline S73 degree 2 poles (-14.4907, 9.7687) (-14.3659, 9.7687) (-14.2354, 9.8522) (-14.2354, 9.9462) knots 0 0 0 1 2 2 2
  spline S74 degree 2 poles (-14.2354, 9.9462) (-14.2354, 9.9956) (-14.2743, 10.0993) (-14.3092, 10.1407) knots 0 0 0 1 2 2 2
  line L72 (-14.1058, 11.0394) -> (-14.1058, 10.913)
  line L73 (-14.1058, 10.913) -> (-14.5336, 10.913)
  spline S75 degree 2 poles (-14.5336, 10.913) (-14.5855, 10.913) (-14.6746, 10.9032) (-14.7014, 10.8887) knots 0 0 0 1 2 2 2
  spline S76 degree 2 poles (-14.7014, 10.8887) (-14.7298, 10.8733) (-14.7573, 10.8181) (-14.7573, 10.7711) knots 0 0 0 1 2 2 2
  spline S77 degree 2 poles (-14.7573, 10.7711) (-14.7573, 10.7241) (-14.7071, 10.6245) (-14.6665, 10.5767) knots 0 0 0 1 2 2 2
  line L74 (-14.6665, 10.5767) -> (-14.1058, 10.5767)
  line L75 (-14.1058, 10.5767) -> (-14.1058, 10.4502)
  line L76 (-14.1058, 10.4502) -> (-15.1503, 10.4502)
  line L77 (-15.1503, 10.4502) -> (-15.1503, 10.5767)
  line L78 (-15.1503, 10.5767) -> (-14.7727, 10.5767)
  spline S78 degree 2 poles (-14.7727, 10.5767) (-14.8238, 10.6334) (-14.8772, 10.7428) (-14.8772, 10.8044) knots 0 0 0 1 2 2 2
  spline S79 degree 2 poles (-14.8772, 10.8044) (-14.8772, 10.9146) (-14.7314, 11.0394) (-14.5928, 11.0394) knots 0 0 0 1 2 2 2
  line L79 (-14.5928, 11.0394) -> (-14.1058, 11.0394)
  spline S80 degree 2 poles (-14.0912, 11.4438) (-14.0912, 11.3408) (-14.2087, 11.225) (-14.3359, 11.225) knots 0 0 0 1 2 2 2
  line L80 (-14.3359, 11.225) -> (-14.7516, 11.225)
  line L81 (-14.7516, 11.225) -> (-14.7516, 11.1399)
  line L82 (-14.7516, 11.1399) -> (-14.8562, 11.1399)
  line L83 (-14.8562, 11.1399) -> (-14.8562, 11.225)
  line L84 (-14.8562, 11.225) -> (-15.0717, 11.225)
  line L85 (-15.0717, 11.225) -> (-15.0717, 11.3514)
  line L86 (-15.0717, 11.3514) -> (-14.8562, 11.3514)
  line L87 (-14.8562, 11.3514) -> (-14.8562, 11.584)
  line L88 (-14.8562, 11.584) -> (-14.7516, 11.584)
  line L89 (-14.7516, 11.584) -> (-14.7516, 11.3514)
  line L90 (-14.7516, 11.3514) -> (-14.3943, 11.3514)
  spline S81 degree 2 poles (-14.3943, 11.3514) (-14.3375, 11.3514) (-14.2751, 11.3554) (-14.2484, 11.3692) knots 0 0 0 1 2 2 2
  spline S82 degree 2 poles (-14.2484, 11.3692) (-14.2249, 11.3805) (-14.2014, 11.4316) (-14.2014, 11.4754) knots 0 0 0 1 2 2 2
  spline S83 degree 2 poles (-14.2014, 11.4754) (-14.2014, 11.5062) (-14.22, 11.5637) (-14.2257, 11.5767) knots 0 0 0 1 2 2 2
  line L91 (-14.2257, 11.5767) -> (-14.2257, 11.584)
  line L92 (-14.2257, 11.584) -> (-14.1123, 11.584)
  spline S84 degree 2 poles (-14.1123, 11.584) (-14.1025, 11.5483) (-14.0912, 11.4754) (-14.0912, 11.4438) knots 0 0 0 1 2 2 2
  spline S85 degree 2 poles (-14.0879, 12.3951) (-14.0879, 12.2865) (-14.1333, 12.1342) (-14.1657, 12.0669) knots 0 0 0 1 2 2 2
  line L93 (-14.1657, 12.0669) -> (-14.3327, 12.0669)
  line L94 (-14.3327, 12.0669) -> (-14.3327, 12.0767)
  spline S86 degree 2 poles (-14.3327, 12.0767) (-14.2711, 12.1423) (-14.203, 12.3084) (-14.203, 12.3854) knots 0 0 0 1 2 2 2
  spline S87 degree 2 poles (-14.203, 12.3854) (-14.203, 12.4956) (-14.2946, 12.6083) (-14.3699, 12.6083) knots 0 0 0 1 2 2 2
  spline S88 degree 2 poles (-14.3699, 12.6083) (-14.4299, 12.6083) (-14.5045, 12.5491) (-14.5231, 12.4851) knots 0 0 0 1 2 2 2
  spline S89 degree 2 poles (-14.5231, 12.4851) (-14.5361, 12.4389) (-14.5539, 12.3619) (-14.5685, 12.3044) knots 0 0 0 1 2 2 2
  spline S90 degree 2 poles (-14.5685, 12.3044) (-14.5823, 12.2525) (-14.6236, 12.1707) (-14.6568, 12.1391) knots 0 0 0 1 2 2 2
  spline S91 degree 2 poles (-14.6568, 12.1391) (-14.69, 12.1083) (-14.7792, 12.0742) (-14.8375, 12.0742) knots 0 0 0 1 2 2 2
  spline S92 degree 2 poles (-14.8375, 12.0742) (-14.9591, 12.0742) (-15.1236, 12.2639) (-15.1236, 12.4105) knots 0 0 0 1 2 2 2
  spline S93 degree 2 poles (-15.1236, 12.4105) (-15.1236, 12.4948) (-15.0904, 12.6439) (-15.0588, 12.7079) knots 0 0 0 1 2 2 2
  line L95 (-15.0588, 12.7079) -> (-14.8999, 12.7079)
  line L96 (-14.8999, 12.7079) -> (-14.8999, 12.6982)
  spline S94 degree 2 poles (-14.8999, 12.6982) (-14.9437, 12.6504) (-15.0085, 12.5013) (-15.0085, 12.4194) knots 0 0 0 1 2 2 2
  spline S95 degree 2 poles (-15.0085, 12.4194) (-15.0085, 12.3271) (-14.9218, 12.2128) (-14.8513, 12.2128) knots 0 0 0 1 2 2 2
  spline S96 degree 2 poles (-14.8513, 12.2128) (-14.7881, 12.2128) (-14.7127, 12.2801) (-14.6957, 12.3433) knots 0 0 0 1 2 2 2
  spline S97 degree 2 poles (-14.6957, 12.3433) (-14.6844, 12.3854) (-14.6552, 12.5078) (-14.643, 12.5483) knots 0 0 0 1 2 2 2
  spline S98 degree 2 poles (-14.643, 12.5483) (-14.6114, 12.6512) (-14.4842, 12.7468) (-14.391, 12.7468) knots 0 0 0 1 2 2 2
  spline S99 degree 2 poles (-14.391, 12.7468) (-14.3319, 12.7468) (-14.2184, 12.699) (-14.1787, 12.6561) knots 0 0 0 1 2 2 2
  spline S100 degree 2 poles (-14.1787, 12.6561) (-14.1349, 12.6083) (-14.0879, 12.4867) (-14.0879, 12.3951) knots 0 0 0 1 2 2 2
  spline S101 degree 2 poles (-14.0888, 13.1982) (-14.0888, 13.0183) (-14.2905, 12.8206) (-14.4769, 12.8206) knots 0 0 0 1 2 2 2
  spline S102 degree 2 poles (-14.4769, 12.8206) (-14.6601, 12.8206) (-14.8772, 13.0126) (-14.8772, 13.1674) knots 0 0 0 1 2 2 2
  spline S103 degree 2 poles (-14.8772, 13.1674) (-14.8772, 13.2371) (-14.8367, 13.3449) (-14.7938, 13.3846) knots 0 0 0 1 2 2 2
  spline S104 degree 2 poles (-14.7938, 13.3846) (-14.7508, 13.4251) (-14.6268, 13.4681) (-14.5369, 13.4681) knots 0 0 0 1 2 2 2
  line L97 (-14.5369, 13.4681) -> (-14.468, 13.4681)
  line L98 (-14.468, 13.4681) -> (-14.468, 12.9486)
  spline S105 degree 2 poles (-14.468, 12.9486) (-14.3375, 12.9486) (-14.199, 13.0799) (-14.199, 13.1966) knots 0 0 0 1 2 2 2
  spline S106 degree 2 poles (-14.199, 13.1966) (-14.199, 13.2379) (-14.2176, 13.3181) (-14.2322, 13.3506) knots 0 0 0 1 2 2 2
  spline S107 degree 2 poles (-14.2322, 13.3506) (-14.2484, 13.3846) (-14.2768, 13.4316) (-14.2897, 13.447) knots 0 0 0 1 2 2 2
  line L99 (-14.2897, 13.447) -> (-14.2897, 13.4543)
  line L100 (-14.2897, 13.4543) -> (-14.152, 13.4543)
  spline S108 degree 2 poles (-14.152, 13.4543) (-14.143, 13.4324) (-14.1171, 13.366) (-14.1098, 13.34) knots 0 0 0 1 2 2 2
  spline S109 degree 2 poles (-14.1098, 13.34) (-14.0993, 13.3036) (-14.0888, 13.2436) (-14.0888, 13.1982) knots 0 0 0 1 2 2 2
  spline S110 degree 2 poles (-14.5644, 13.3449) (-14.6155, 13.3433) (-14.69, 13.3222) (-14.7152, 13.3019) knots 0 0 0 1 2 2 2
  spline S111 degree 2 poles (-14.7152, 13.3019) (-14.7435, 13.2801) (-14.7735, 13.2112) (-14.7735, 13.1601) knots 0 0 0 1 2 2 2
  spline S112 degree 2 poles (-14.7735, 13.1601) (-14.7735, 13.1099) (-14.7435, 13.0394) (-14.7144, 13.0102) knots 0 0 0 1 2 2 2
  spline S113 degree 2 poles (-14.7144, 13.0102) (-14.6844, 12.9818) (-14.6123, 12.9527) (-14.5644, 12.9486) knots 0 0 0 1 2 2 2
  line L101 (-14.5644, 12.9486) -> (-14.5644, 13.3449)
  line L102 (-14.1058, 14.1852) -> (-14.1058, 14.0588)
  line L103 (-14.1058, 14.0588) -> (-14.5336, 14.0588)
  spline S114 degree 2 poles (-14.5336, 14.0588) (-14.5855, 14.0588) (-14.6746, 14.0491) (-14.7014, 14.0345) knots 0 0 0 1 2 2 2
  spline S115 degree 2 poles (-14.7014, 14.0345) (-14.7298, 14.0191) (-14.7573, 13.964) (-14.7573, 13.917) knots 0 0 0 1 2 2 2
  spline S116 degree 2 poles (-14.7573, 13.917) (-14.7573, 13.87) (-14.7071, 13.7703) (-14.6665, 13.7225) knots 0 0 0 1 2 2 2
  line L104 (-14.6665, 13.7225) -> (-14.1058, 13.7225)
  line L105 (-14.1058, 13.7225) -> (-14.1058, 13.5961)
  line L106 (-14.1058, 13.5961) -> (-14.8562, 13.5961)
  line L107 (-14.8562, 13.5961) -> (-14.8562, 13.7225)
  line L108 (-14.8562, 13.7225) -> (-14.7727, 13.7225)
  spline S117 degree 2 poles (-14.7727, 13.7225) (-14.8238, 13.7793) (-14.8772, 13.8887) (-14.8772, 13.9502) knots 0 0 0 1 2 2 2
  spline S118 degree 2 poles (-14.8772, 13.9502) (-14.8772, 14.0605) (-14.7314, 14.1852) (-14.5928, 14.1852) knots 0 0 0 1 2 2 2
  line L109 (-14.5928, 14.1852) -> (-14.1058, 14.1852)
  spline S119 degree 2 poles (-14.0879, 14.5653) (-14.0879, 14.4899) (-14.1285, 14.3595) (-14.1511, 14.3165) knots 0 0 0 1 2 2 2
  line L110 (-14.1511, 14.3165) -> (-14.293, 14.3165)
  line L111 (-14.293, 14.3165) -> (-14.293, 14.323)
  spline S120 degree 2 poles (-14.293, 14.323) (-14.28, 14.3392) (-14.2492, 14.383) (-14.2322, 14.4194) knots 0 0 0 1 2 2 2
  spline S121 degree 2 poles (-14.2322, 14.4194) (-14.2168, 14.4511) (-14.1941, 14.5288) (-14.1941, 14.5702) knots 0 0 0 1 2 2 2
  spline S122 degree 2 poles (-14.1941, 14.5702) (-14.1941, 14.6002) (-14.2079, 14.669) (-14.2192, 14.6852) knots 0 0 0 1 2 2 2
  spline S123 degree 2 poles (-14.2192, 14.6852) (-14.2346, 14.7087) (-14.2695, 14.7298) (-14.3051, 14.7298) knots 0 0 0 1 2 2 2
  spline S124 degree 2 poles (-14.3051, 14.7298) (-14.3497, 14.7298) (-14.3959, 14.6812) (-14.4113, 14.6188) knots 0 0 0 1 2 2 2
  spline S125 degree 2 poles (-14.4113, 14.6188) (-14.417, 14.5945) (-14.4332, 14.5167) (-14.4421, 14.4835) knots 0 0 0 1 2 2 2
  spline S126 degree 2 poles (-14.4421, 14.4835) (-14.4672, 14.3976) (-14.5709, 14.3198) (-14.6447, 14.3198) knots 0 0 0 1 2 2 2
  spline S127 degree 2 poles (-14.6447, 14.3198) (-14.7468, 14.3198) (-14.874, 14.4729) (-14.874, 14.5993) knots 0 0 0 1 2 2 2
  spline S128 degree 2 poles (-14.874, 14.5993) (-14.874, 14.6617) (-14.8432, 14.7882) (-14.8197, 14.8311) knots 0 0 0 1 2 2 2
  line L112 (-14.8197, 14.8311) -> (-14.6844, 14.8311)
  line L113 (-14.6844, 14.8311) -> (-14.6844, 14.8246)
  spline S129 degree 2 poles (-14.6844, 14.8246) (-14.7233, 14.776) (-14.7678, 14.6577) (-14.7678, 14.5969) knots 0 0 0 1 2 2 2
  spline S130 degree 2 poles (-14.7678, 14.5969) (-14.7678, 14.5345) (-14.7152, 14.4486) (-14.6625, 14.4486) knots 0 0 0 1 2 2 2
  spline S131 degree 2 poles (-14.6625, 14.4486) (-14.6147, 14.4486) (-14.5685, 14.4997) (-14.5539, 14.5564) knots 0 0 0 1 2 2 2
  spline S132 degree 2 poles (-14.5539, 14.5564) (-14.5466, 14.584) (-14.532, 14.6536) (-14.5231, 14.6917) knots 0 0 0 1 2 2 2
  spline S133 degree 2 poles (-14.5231, 14.6917) (-14.502, 14.7744) (-14.4056, 14.8587) (-14.3221, 14.8587) knots 0 0 0 1 2 2 2
  spline S134 degree 2 poles (-14.3221, 14.8587) (-14.2735, 14.8587) (-14.1876, 14.8206) (-14.156, 14.7833) knots 0 0 0 1 2 2 2
  spline S135 degree 2 poles (-14.156, 14.7833) (-14.1228, 14.7436) (-14.0879, 14.6423) (-14.0879, 14.5653) knots 0 0 0 1 2 2 2
  spline S136 degree 2 poles (-14.481, 15.5929) (-14.2913, 15.5929) (-14.0847, 15.4105) (-14.0847, 15.2582) knots 0 0 0 1 2 2 2
  spline S137 degree 2 poles (-14.0847, 15.2582) (-14.0847, 15.1018) (-14.2978, 14.9227) (-14.481, 14.9227) knots 0 0 0 1 2 2 2
  spline S138 degree 2 poles (-14.481, 14.9227) (-14.669, 14.9227) (-14.8772, 15.1075) (-14.8772, 15.2582) knots 0 0 0 1 2 2 2
  spline S139 degree 2 poles (-14.8772, 15.2582) (-14.8772, 15.4105) (-14.6698, 15.5929) (-14.481, 15.5929) knots 0 0 0 1 2 2 2
  spline S140 degree 2 poles (-14.481, 15.4624) (-14.6268, 15.4624) (-14.7687, 15.3562) (-14.7687, 15.2582) knots 0 0 0 1 2 2 2
  spline S141 degree 2 poles (-14.7687, 15.2582) (-14.7687, 15.1601) (-14.6268, 15.0532) (-14.481, 15.0532) knots 0 0 0 1 2 2 2
  spline S142 degree 2 poles (-14.481, 15.0532) (-14.3392, 15.0532) (-14.1933, 15.1601) (-14.1933, 15.2582) knots 0 0 0 1 2 2 2
  spline S143 degree 2 poles (-14.1933, 15.2582) (-14.1933, 15.3554) (-14.3367, 15.4624) (-14.481, 15.4624) knots 0 0 0 1 2 2 2
  line L114 (-14.7208, 16.1204) -> (-14.7208, 16.1139)
  spline S144 degree 2 poles (-14.7208, 16.1139) (-14.7249, 16.0993) (-14.7265, 16.0677) (-14.7265, 16.0459) knots 0 0 0 1 2 2 2
  spline S145 degree 2 poles (-14.7265, 16.0459) (-14.7265, 15.9948) (-14.6819, 15.8943) (-14.6382, 15.8489) knots 0 0 0 1 2 2 2
  line L115 (-14.6382, 15.8489) -> (-14.1058, 15.8489)
  line L116 (-14.1058, 15.8489) -> (-14.1058, 15.7225)
  line L117 (-14.1058, 15.7225) -> (-14.8562, 15.7225)
  line L118 (-14.8562, 15.7225) -> (-14.8562, 15.8489)
  line L119 (-14.8562, 15.8489) -> (-14.7443, 15.8489)
  spline S146 degree 2 poles (-14.7443, 15.8489) (-14.8059, 15.9178) (-14.8562, 16.0207) (-14.8562, 16.0694) knots 0 0 0 1 2 2 2
  spline S147 degree 2 poles (-14.8562, 16.0694) (-14.8562, 16.0888) (-14.8546, 16.1083) (-14.8521, 16.1204) knots 0 0 0 1 2 2 2
  line L120 (-14.8521, 16.1204) -> (-14.7208, 16.1204)
  point P0 (0, 0)
  constraints: 4 other
extrude "Extrusion20" cut sketch "Esquisse16" against normal blind 0.01